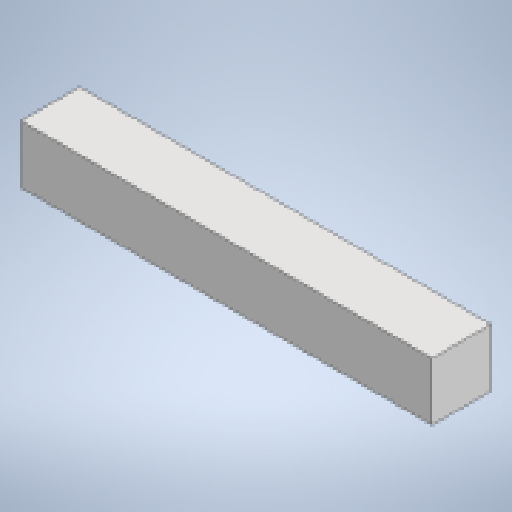
# Autodesk Inventor part: 부품73
Saved by Autodesk Inventor 2024 (Build 280153000, 153)
## iProperties
Created: 2024-09-08
Part Number: 부품73
Material: 일반
Document SubType Name: Modeling
Designer: Eungang
Density: 1 g/cm^3
Appearance: 기본값
Author: Eungang
Autodesk Inventor part; units mm, degrees
ref_plane "YZ Plane" through (0, 0, 0) normal (1, 0, 0) x (0, 1, 0)
ref_plane "XZ Plane" through (0, 0, 0) normal (0, 1, 0) x (-1, 0, 0)
ref_plane "XY Plane" through (0, 0, 0) normal (0, 0, 1) x (1, 0, 0)
sketch "스케치1" plane through (0, 0, 0) normal (0, 0, 1) x (1, 0, 0)
  circle A0 centre (14.75, -25.8408) radius 14.2 projected
  line L0 (41.95, 5.9) -> (41.95, -57.9408) projected
  line L1 (-41.95, 5.9) -> (41.95, 5.9) projected
  line L2 (-41.95, -57.9408) -> (-41.95, 5.9) projected
  line L3 (41.95, -57.9408) -> (-41.95, -57.9408) projected
  line L4 (-41.95, 5.9) -> (0, 5.9)
  line L5 (0, 5.9) -> (0, 0)
  line L6 (0, 0) -> (-41.95, 0)
  line L7 (-41.95, 0) -> (-41.95, 5.9)
  line L8 (-41.95, 0) -> (0, 0)
  line L9 (0, 0) -> (0, 2.95)
  line L10 (0, 2.95) -> (-41.95, 2.95)
  line L11 (-41.95, 2.95) -> (-41.95, 0)
  constraints: 16 end point, 4 parallel, 2 horizontal, 2 perpendicular, 1 midpoint
extrude "돌출1" add sketch "스케치1" along normal blind 6 contours L5 L6 L2 L10
sketch "스케치2" plane through (-41.95, 0, 0) normal (-1, 0, 0) x (0, 0, 1)
  point P0 (0, 0)
ref_plane "작업 평면1" through (0, 0, 0) normal (0, 0, 1) x (1, 0, 0)
sketch "스케치3" plane through (0, 0, 0) normal (0, 0, 1) x (1, 0, 0)
  point P0 (0, 0)
sketch "스케치4" plane through (0, 0, 0) normal (0, 0, 1) x (1, 0, 0)
  circle A0 centre (14.75, -25.8408) radius 14.2 projected
  line L0 (41.95, 5.9) -> (41.95, -57.9408) projected
  line L1 (-41.95, 5.9) -> (41.95, 5.9) projected
  line L2 (-41.95, -57.9408) -> (-41.95, 5.9) projected
  line L3 (41.95, -57.9408) -> (-41.95, -57.9408) projected
  line L4 (-41.95, 5.9) -> (0, 5.9)
  line L5 (0, 5.9) -> (0, 2.95)
  line L6 (0, 2.95) -> (-41.95, 2.95)
  line L7 (-41.95, 2.95) -> (-41.95, 5.9)
  point P0 (0, 0)
  point P1 (0, 5.9)
  constraints: 8 end point, 2 parallel, 1 horizontal, 1 perpendicular
extrude "돌출2" add sketch "스케치4" along normal blind 3 contours L5 L6 L2 L1
